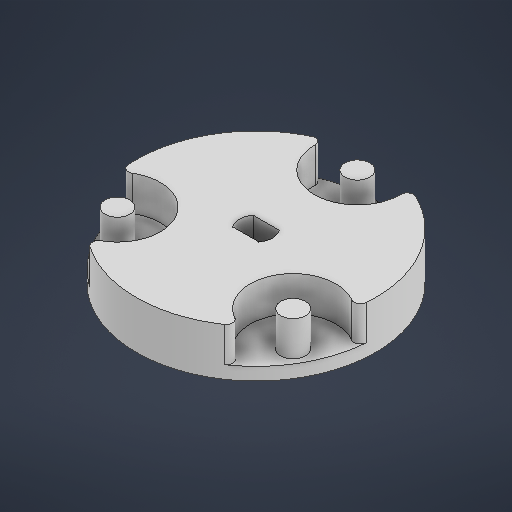
# Autodesk Inventor part: gewindeding
Saved by Autodesk Inventor 2026.2 (Build 302298000, 298)
## iProperties
Created: 2026-03-16
Part Number: gewindeding
Material: Generic
Document SubType Name: Modeling
Designer: Cobble
Density: 1 g/cm^3
Appearance: Default
Author: Cobble
Autodesk Inventor part; units mm, degrees
ref_plane "YZ Plane" through (0, 0, 0) normal (1, 0, 0) x (0, 1, 0)
ref_plane "XZ Plane" through (0, 0, 0) normal (0, 1, 0) x (-1, 0, 0)
ref_plane "XY Plane" through (0, 0, 0) normal (0, 0, 1) x (1, 0, 0)
sketch "Sketch1" plane through (0, 0, 0) normal (0, 0, 1) x (1, 0, 0)
  circle A0 centre (0, 0) radius 6.75
  circle A1 centre (0, 0) radius 1.95
  line L0 (0, 0) -> (0, -16)
  circle A2 centre (-13.8564, -24) radius 6.75
  circle A3 centre (-13.8564, -24) radius 1.95
  line L1 (-13.8564, -24) -> (0, -16) construction
  circle A4 centre (13.8564, -24) radius 6.75
  circle A5 centre (13.8564, -24) radius 1.95
  line L2 (13.8564, -24) -> (0, -16)
  circle A6 centre (0, -16) radius 18.85
  circle A7 centre (0, -16) radius 1.05 construction
  circle A8 centre (0, -16) radius 2.6
  line L3 (-2.7713, -14.4) -> (2.7713, -14.4)
  line L4 (2.7713, -14.4) -> (2.7713, -17.6)
  line L5 (2.7713, -17.6) -> (-2.7713, -17.6)
  line L6 (-2.7713, -17.6) -> (-2.7713, -14.4)
  line L7 (-2.7713, -14.4) -> (2.7713, -17.6) construction
  line L8 (2.7713, -14.4) -> (-2.7713, -17.6) construction
  point P0 (18.5801, -19.1783)
  point P1 (6.5376, 1.68)
  point P2 (-6.5376, 1.68)
  point P3 (-18.5801, -19.1783)
  point P4 (-12.0425, -30.5017)
  point P5 (12.0425, -30.5017)
  point P6 (-2.0494, -17.6)
  point P7 (-2.0494, -14.4)
  point P8 (2.0494, -14.4)
  point P9 (2.0494, -17.6)
  dimension "d0" = 13.5
  dimension "d1" = 3.9
  dimension "d2" = 16
  dimension "d5" = 360
  dimension "d12" = 2.1
  dimension "d14" = 37.7
  dimension "d15" = 5.2
  dimension "d21" = 3.2
  constraints: 18 end point, 10 coincident, 9 centre point, 3 point on line, 2 midpoint, 2 parallel, 1 horizontal, 1 perpendicular, 1 vertical, 20 other
  measures "d0" diameter of A0
  measures "d1" diameter of A1
  measures "d2" distance of L0.start L0.end
  measures "d12" diameter of A7
  measures "d14" diameter of A6
  measures "d15" diameter of A8
  measures "d21" distance of L3.end L4.end
extrude "Extrusion1" add sketch "Sketch1" along normal blind 5.5 contours A1 | A0 A6 A4 L2 L4 L3 A8 L0 | L0 A8 L3 L6 L5 L2 A4 A6 A2 A0 | A8 L3 L0 | L0 L3 A8 | A5 | L3 L4 L2 A8 | A8 L5 L6 L3 | L5 A8 | L5 A8 L2 | A3
extrude "Extrusion2" add sketch "Sketch1" against normal blind 2 contours A1 | A0 A6 | A0 A6 A4 L2 L4 L3 A8 L0 | L0 A8 L3 L6 L5 L2 A4 A6 A2 A0 | A8 L3 L0 | L0 L3 A8 | A2 A6 | A5 | A6 A4 | L3 L4 L2 A8 | A8 L5 L6 L3 | L5 A8 | L5 A8 L2 | A3 picked at (3.5494, 1.6258) picked at (-17.0724, -21.7739) picked at (17.0771, -21.7793)
fillet "Fillet1" radius 1 6 edges at (-12.0425, -30.5017, 2.75) (-18.5801, -19.1783, 2.75) (18.5801, -19.1783, 2.75) (12.0425, -30.5017, 2.75) (6.5376, 1.68, 2.75) (-6.5376, 1.68, 2.75)
body "Solid1"
